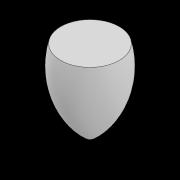
# Autodesk Inventor part: McCrea_eva_walle
Saved by Autodesk Inventor 2021 (Build 250183000, 183)
## iProperties
Created: 2022-01-17
Part Number: McCrea_eva_walle
Material: Generic
Document SubType Name: Modeling
Designer: student
Density: 1 g/cm^3
Appearance: Default
Author: student
Autodesk Inventor part; units mm, degrees
ref_plane "YZ Plane" through (0, 0, 0) normal (1, 0, 0) x (0, 1, 0)
ref_plane "XZ Plane" through (0, 0, 0) normal (0, 1, 0) x (-1, 0, 0)
ref_plane "XY Plane" through (0, 0, 0) normal (0, 0, 1) x (1, 0, 0)
sketch "Sketch1" plane through (0, 0, 0) normal (0, 0, 1) x (1, 0, 0)
  line L0 (0, -51) -> (0, 59)
  line L1 (0, 59) -> (-40, 59)
  line L2 (0, -51) -> (-5, -51)
  arc A0 (-40, 59) -> (-5, -51) centre (66.7335, 32.3925) ccw
  point P0 (0, 0)
  dimension "d0" = 40
  dimension "d1" = 5
  dimension "d2" = 110
  dimension "d4" = 110
  constraints: 6 end point, 2 horizontal, 2 point on circle, 1 centre point, 1 vertical
  measures "d0" distance of L0.end L1.end
  measures "d1" distance of L0.start L2.end
  measures "d2" radius of A0
  measures "d4" distance of L0.start L0.end
revolve "Revolution1" add sketch "Sketch1" angle 360 about axis through (0, -51, 0) along (0, 1, 0)
body "Solid1"
